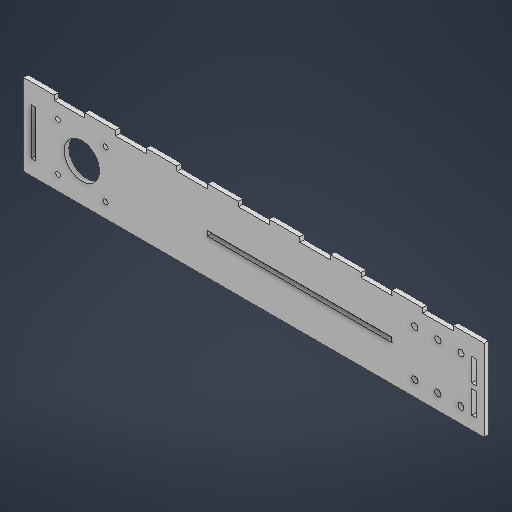
# Autodesk Inventor part: Sideboard
Saved by Autodesk Inventor 2027 (Build 310192000, 192)
## iProperties
Created: 2026-05-09
Part Number: Sideboard
Material: Generic
Document SubType Name: Modeling
Designer: alexy
Density: 1 g/cm^3
Appearance: Default
Author: alexy
Autodesk Inventor part; units mm, degrees
ref_plane "YZ Plane" through (0, 0, 0) normal (1, 0, 0) x (0, 1, 0)
ref_plane "XZ Plane" through (0, 0, 0) normal (0, 1, 0) x (-1, 0, 0)
ref_plane "XY Plane" through (0, 0, 0) normal (0, 0, 1) x (1, 0, 0)
sketch "Sketch1" plane through (0, 0, 0) normal (0, 0, 1) x (1, 0, 0)
  line L0 (0, 0) -> (300, 0)
  line L1 (300, 0) -> (300, 50)
  line L2 (300, 50) -> (0, 50)
  line L3 (0, 50) -> (0, 0)
  circle A0 centre (22.6, 40.5) radius 1.55
  circle A1 centre (22.6, 9.5) radius 1.55
  circle A2 centre (53.6, 40.5) radius 1.55
  circle A3 centre (53.6, 9.5) radius 1.55
  circle A4 centre (38.1, 25) radius 11.5
  line L4 (120, 26.55) -> (240, 26.55)
  line L5 (240, 26.55) -> (240, 23.45)
  line L6 (240, 23.45) -> (120, 23.45)
  line L7 (120, 23.45) -> (120, 26.55)
  line L8 (0, 50) -> (19.6145, 50)
  line L9 (0, 50) -> (20, 50)
  line L10 (20, 50) -> (20, 53)
  line L11 (20, 53) -> (0, 53)
  line L12 (0, 53) -> (0, 50)
  line L13 (40, 50) -> (60, 50)
  line L14 (40, 50) -> (60, 50)
  line L15 (60, 50) -> (60, 53)
  line L16 (60, 53) -> (40, 53)
  line L17 (40, 53) -> (40, 50)
  line L18 (80, 50) -> (100, 50)
  line L19 (80, 50) -> (100, 50)
  line L20 (100, 50) -> (100, 53)
  line L21 (100, 53) -> (80, 53)
  line L22 (80, 53) -> (80, 50)
  line L23 (120, 50) -> (140, 50)
  line L24 (120, 50) -> (140, 50)
  line L25 (140, 50) -> (140, 53)
  line L26 (140, 53) -> (120, 53)
  line L27 (120, 53) -> (120, 50)
  line L28 (160, 50) -> (180, 50)
  line L29 (160, 50) -> (180, 50)
  line L30 (180, 50) -> (180, 53)
  line L31 (180, 53) -> (160, 53)
  line L32 (160, 53) -> (160, 50)
  line L33 (200, 50) -> (217.051, 50)
  line L34 (200, 50) -> (220, 50)
  line L35 (220, 50) -> (220, 53)
  line L36 (220, 53) -> (200, 53)
  line L37 (200, 53) -> (200, 50)
  line L38 (260, 50) -> (260, 53)
  line L39 (260, 53) -> (240, 53)
  line L40 (240, 53) -> (240, 50)
  line L41 (240, 50) -> (257.051, 50)
  line L42 (240, 50) -> (260, 50)
  line L43 (300, 50) -> (300, 53)
  line L44 (300, 53) -> (280, 53)
  line L45 (280, 53) -> (280, 50)
  line L46 (280, 50) -> (297.051, 50)
  line L47 (280, 50) -> (300, 50)
  line L48 (8.1, 10) -> (5, 10)
  line L49 (5, 10) -> (5, 40)
  line L50 (5, 40) -> (8.1, 40)
  line L51 (8.1, 40) -> (8.1, 10)
  line L52 (8.1, 10) -> (5, 40) construction
  line L53 (5, 10) -> (8.1, 40) construction
  circle A5 centre (285, 10) radius 2.05
  circle A6 centre (270, 10) radius 2.05
  circle A7 centre (285, 40) radius 2.05
  circle A8 centre (270, 40) radius 2.05
  circle A9 centre (255, 40) radius 2.05
  circle A10 centre (255, 10) radius 2.05
  line L54 (291.9, 23.45) -> (295, 23.45)
  line L55 (295, 23.45) -> (295, 8.45)
  line L56 (295, 8.45) -> (291.9, 8.45)
  line L57 (291.9, 8.45) -> (291.9, 23.45)
  line L58 (291.9, 26.55) -> (295, 26.55)
  line L59 (295, 26.55) -> (295, 41.55)
  line L60 (295, 41.55) -> (291.9, 41.55)
  line L61 (291.9, 41.55) -> (291.9, 26.55)
  point P0 (6.55, 25)
  point P1 (5, 25)
  point P2 (8.1, 25)
  point P3 (120, 25)
  dimension "d1" = 3.1
  dimension "d2" = 3.1
  dimension "d3" = 3.1
  dimension "d4" = 3.1
  dimension "d5" = 31
  dimension "d7" = 23
  dimension "d8" = 15.5
  dimension "d9" = 15.5
  dimension "d10" = 50
  dimension "d11" = 31
  dimension "d12" = 3.1
  dimension "d13" = 25
  dimension "d32" = 20
  dimension "d33" = 3
  dimension "d34" = 20
  dimension "d35" = 3
  dimension "d36" = 20
  dimension "d37" = 3
  dimension "d38" = 20
  dimension "d39" = 3
  dimension "d40" = 20
  dimension "d41" = 3
  dimension "d42" = 20
  dimension "d43" = 20
  dimension "d44" = 20
  dimension "d45" = 20
  dimension "d46" = 20
  dimension "d47" = 3
  dimension "d48" = 20
  dimension "d49" = 3
  dimension "d50" = 20
  dimension "d51" = 3
  dimension "d52" = 20
  dimension "d53" = 20
  dimension "d54" = 300
  dimension "d55" = 3.1
  dimension "d56" = 5
  dimension "d57" = 15
  dimension "d58" = 30
  dimension "d59" = 120
  dimension "d60" = 60
  dimension "d63" = 4.1
  dimension "d64" = 4.1
  dimension "d65" = 4.1
  dimension "d66" = 4.1
  dimension "d67" = 4.1
  dimension "d68" = 4.1
  dimension "d69" = 15
  dimension "d70" = 15
  dimension "d71" = 10
  dimension "d72" = 10
  dimension "d73" = 15
  dimension "d74" = 3.1
  dimension "d75" = 15
  dimension "d77" = 15
  dimension "d78" = 5
  constraints: 124 end point, 26 parallel, 21 horizontal, 17 horizontal alignment, 13 perpendicular, 11 centre point, 8 vertical alignment, 5 midpoint
  measures "d1" diameter of A0
  measures "d2" diameter of A1
  measures "d3" diameter of A2
  measures "d4" diameter of A3
  measures "d5" distance of A1.centre A3.centre
  measures "d7" diameter of A4
  measures "d8" horizontal distance of A0.centre A4.centre
  measures "d9" horizontal distance of A4.centre A3.centre
  measures "d10" distance of L0.end L1.end
  measures "d11" distance of A3.centre A2.centre
  measures "d12" distance of L6.end L4.start
  measures "d13" distance from line of L0 A4.centre
  measures "d32" distance of L11.end L10.end
  measures "d33" distance of L11.end L2.end
  measures "d34" distance of L16.end L15.end
  measures "d35" distance of L16.end L17.end
  measures "d36" distance of L21.end L20.end
  measures "d37" distance of L21.end L22.end
  measures "d38" distance of L26.end L25.end
  measures "d39" distance of L26.end L27.end
  measures "d40" distance of L31.end L30.end
  measures "d41" distance of L31.end L32.end
  measures "d42" distance of L16.end L10.end
  measures "d43" distance of L15.end L21.end
  measures "d44" distance of L20.end L26.end
  measures "d45" distance of L25.end L31.end
  measures "d46" distance of L36.end L36.start
  measures "d47" distance of L36.end L34.start
  measures "d48" distance of L40.start L38.end
  measures "d49" distance of L40.start L40.end
  measures "d50" distance of L45.start L43.end
  measures "d51" distance of L45.start L46.start
  measures "d52" distance of L40.start L36.start
  measures "d53" distance of L38.end L45.start
  measures "d54" distance of L0.end L0.start
  measures "d55" distance of L49.end L50.end
  measures "d56" distance between parallel lines of L3 L49
  measures "d57" distance of point (5, 25) L49.end
  measures "d58" distance of point (8.1, 25) A4.centre
  measures "d59" distance of L5.end L6.end
  measures "d60" distance between parallel lines of L1 L5
  measures "d63" diameter of A5
  measures "d64" diameter of A6
  measures "d65" diameter of A7
  measures "d66" diameter of A8
  measures "d67" diameter of A9
  measures "d68" diameter of A10
  measures "d69" distance of A6.centre A5.centre
  measures "d70" distance of A10.centre A6.centre
  measures "d71" distance from line of L0 A5.centre
  measures "d72" distance from line of L2 A7.centre
  measures "d73" distance from line of L1 A5.centre
  measures "d74" distance of L55.end L56.end
  measures "d75" distance of L54.end L55.end
  measures "d77" distance of L58.end L59.end
  measures "d78" distance from line of L1 L59.end
extrude "Extrusion1" add sketch "Sketch1" along normal blind 3
body "Solid1"
